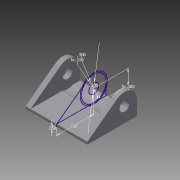
# Autodesk Inventor part: LegHolderV3
Saved by Autodesk Inventor 2014 (Build 180170000, 170)
## iProperties
Created: 2014-04-25
Part Number: LegHolderV3
Material: Generic
Document SubType Name: Modeling
Designer: Max
Density: 1 g/cm^3
Appearance: Default
Author: Max
Autodesk Inventor part; units mm, degrees
ref_plane "YZ Plane" through (0, 0, 0) normal (1, 0, 0) x (0, 1, 0)
ref_plane "XZ Plane" through (0, 0, 0) normal (0, 1, 0) x (-1, 0, 0)
ref_plane "XY Plane" through (0, 0, 0) normal (0, 0, 1) x (1, 0, 0)
sketch "Sketch1" plane through (0, 0, 0) normal (1, 0, 0) x (0, 1, 0)
  circle A0 centre (0, 0) radius 2.54
  circle A1 centre (0, 0) radius 6.35
  line L0 (-7.62, -6.35) -> (-7.62, 19.05)
  line L1 (-7.62, 19.05) -> (-6.35, 19.05)
  line L2 (-6.35, 19.05) -> (5.08, 3.81)
  line L3 (-7.62, -6.35) -> (0, -6.35)
  line L4 (-6.35, 19.05) -> (-6.35, -6.35)
  circle A2 centre (0, 0) radius 6.985
  dimension "d0" = 5.08
  dimension "d1" = 12.7
  dimension "d2" = 7.62
  dimension "d3" = 19.05
  dimension "d4" = 1.27
  dimension "d9" = 13.97
  constraints: 10 end point, 3 centre point, 3 coincident, 2 perpendicular, 2 point on circle, 2 tangent, 1 horizontal, 1 point on line, 1 vertical
  measures "d0" diameter of A0
  measures "d1" diameter of A1
  measures "d2" distance from line of A1.centre L0
  measures "d3" distance from line of point (0, 0) L1
  measures "d4" distance of L0.end L1.end
  measures "d9" diameter of A2
extrude "Extrusion1" add sketch "Sketch1" along normal mid plane 31.75 contours A1 | A1 L4 A2 L2 | L3 A2 L4 A1 | L4 A2 | A2 L4 L2 | L3 L4 A2 | A2 L4 L3 L0 L1
extrude "Extrusion2" cut sketch "Sketch1" along normal mid plane 26.67 contours A0 | A1 | A1 L2 A2 L3 | A1 L4 A2 L2 | L3 A2 L4 A1 | L4 A2 | A2 L4 L2 | L3 L4 A2
equation "\"d9\" = d1 + d4"
body "Solid1"
